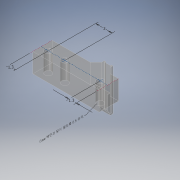
# Autodesk Inventor part: Mid_test
Saved by Autodesk Inventor 2020 (Build 240168000, 168)
## iProperties
Created: 2019-02-01
Part Number: Mid_test
Material: 일반
Document SubType Name: Modeling
Designer: Jeong Ji Hoon
Density: 1 g/cm^3
Appearance: 연회색 반사
Author: Jeong Ji Hoon
## iProperties of the stored document _3D 인쇄.ipt
Created: 2019-11-29
Part Number: _3D 인쇄
Material: 일반
Document SubType Name: Modeling
Designer: Knowblesse
Density: 1 g/cm^3
Appearance: 기본값
Author: Knowblesse
Autodesk Inventor part; units mm, degrees
ref_plane "YZ Plane" through (0, 0, 0) normal (1, 0, 0) x (0, 1, 0)
ref_plane "XZ Plane" through (0, 0, 0) normal (0, 1, 0) x (-1, 0, 0)
ref_plane "XY Plane" through (0, 0, 0) normal (0, 0, 1) x (1, 0, 0)
sketch "스케치1" plane through (0, 0, 0) normal (0, 1, 0) x (-1, 0, 0)
  line L0 (0, 0) -> (12, 0)
  line L1 (12, 0) -> (12, -4)
  line L2 (12, -4) -> (0, -4)
  line L3 (0, -4) -> (0, 0)
  dimension "d0" = 12
  dimension "d1" = 4
  constraints: 8 end point, 2 parallel, 1 horizontal, 1 perpendicular
  measures "d0" distance of L1.end L2.end
  measures "d1" distance of L0.end L1.end
extrude "돌출1" add sketch "스케치1" along normal blind 3.5
sketch "스케치2" plane through (0, 3.5, 0) normal (0, 1, 0) x (1, 0, 0)
  line L0 (0, 0) -> (0, 4) construction
  line L1 (0, 2) -> (-12, 2) construction
  line L2 (-12, 4) -> (-12, 0) construction
  point P0 (-1.3, 2)
  point P1 (-7.7, 2)
  point P2 (-10.7, 2)
  dimension "d59" = 1.3
  dimension "d60" = 3
  dimension "d62" = 1.3
  constraints: 3 point on line, 2 end point, 2 midpoint
  measures "d59" distance from line of L2 point (-10.7, 2)
  measures "d60" distance of point (-10.7, 2) point (-7.7, 2)
  measures "d62" distance from line of L0 point (-1.3, 2)
hole "구멍1" at (-10.7, 3.5, -2) at (-1.3, 3.5, -2) direction (0, -1, 0) diameter 1.2 end through all
hole "구멍2" at (-7.7, 3.5, -2) direction (0, -1, 0) diameter 1.2 end through all
sketch "스케치11" plane through (0, 0, -4) normal (0, 0, -1) x (-1, 0, 0)
  line L0 (0, 0) -> (12, 0) projected
  line L1 (0, 0) -> (0, 3.5) projected
  line L2 (12, 3.5) -> (0, 3.5) projected
  line L3 (12, 0) -> (12, 3.5) projected
  line L4 (12, 3.5) -> (0, 3.5) projected
  line L5 (2.5, 3.5) -> (4.1, 3.5)
  line L6 (4.1, 3.5) -> (4.1, -4)
  line L7 (4.1, -4) -> (2.5, -4)
  line L8 (2.5, -4) -> (2.5, 3.5)
  dimension "d99" = 1.6
  dimension "d100" = 4
  dimension "d124" = 2.5
  constraints: 8 end point, 2 parallel, 1 horizontal, 1 perpendicular, 1 point on line
  measures "d99" distance of L6.end L7.end
  measures "d100" distance between parallel lines of L0 L7
  measures "d124" distance between parallel lines of L8 L1
extrude "돌출9" add sketch "스케치11" along normal blind 1.5 contours L8 L2 L6 L0 | L0 L6 L7 L8
chamfer "모따기6" distance 1 angle 45 2 edges at (-2.5, 1.75, -4) (-4.1, 1.75, -4)
chamfer "모따기7" distance 0.5 angle 45 2 edges at (-2.5, 0, -4.5) (-4.1, 0, -4.5)
sketch "스케치12" plane through (0, 0, -5.5) normal (0, 0, -1) x (-1, 0, 0)
  line L0 (4.1, 3.5) -> (2.5, 3.5) projected
  line L1 (2.5, 3.5) -> (2.5, -4) projected
  line L2 (2.5, -4) -> (4.1, -4) projected
  line L3 (4.1, -4) -> (4.1, 3.5) projected
  line L4 (2.8, -4) -> (2.8, 3.5)
  line L5 (12, 3.5) -> (0, 3.5) projected
  line L6 (3.8, 3.5) -> (3.8, -4)
  line L7 (2.5, -4) -> (4.1, -4) projected
  point P0 (0, 0)
  point P1 (3.8, -4)
  dimension "d110" = 1
  dimension "d111" = 0.3
  dimension "d112" = 0.3
  constraints: 4 end point, 4 point on line, 2 perpendicular
  measures "d110" distance between parallel lines of L6 L4
  measures "d111" distance between parallel lines of L1 L4
  measures "d112" distance between parallel lines of L3 L6
extrude "돌출10" cut sketch "스케치12" against normal blind 0.2 contours L6 L2 L4 L0
sketch "스케치13" plane through (0, 0, -4) normal (0, 0, 1) x (1, 0, 0)
  line L0 (-4.6, 0) -> (-2, 0) projected
  line L1 (-4.1, -0.5) -> (-4.6, 0) projected
  line L2 (-4.1, -4) -> (-4.1, -0.5) projected
  line L3 (-2.5, -4) -> (-4.1, -4) projected
  line L4 (-2.5, -0.5) -> (-2.5, -4) projected
  line L5 (-2, 0) -> (-2.5, -0.5) projected
  point P0 (0, 0)
extrude "돌출11" cut sketch "스케치13" against normal blind 0.5
chamfer "모따기8" distance 0.5 distance2 1 1 edges at (-3.3, -4, -4.5) measured on face at (-3.3, -4, -5)
sketch "스케치14" plane through (-12, 0, 0) normal (0, 0, 1) x (1, 0, 0)
  line L0 (12, 0) -> (0, 0) projected
  line L1 (12, 0) -> (12, 3.5) projected
  line L2 (0, 3.5) -> (12, 3.5) projected
  line L3 (0, 0) -> (0, 3.5) projected
extrude "돌출12" cut sketch "스케치14" against normal blind 0.5
equation "\"d111\" = d112"
equation "\"G23_F\" = 0.65"
equation "\"G23_M\" = 0.67"
equation "\"Screw_F\" = 1.3"
equation "\"Screw_M\" = 1.6"
